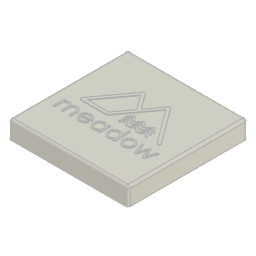
MeadowBox (Autodesk Fusion 360 design; units mm, degrees)
Autodesk Fusion 360 part; units mm, degrees
note: some values were not read from the file. Set by a fixed rule: which sketch regions a step uses.
(part 1 of 2)
sketch "Floor" plane through (0, 0, 0) normal (0, 0, 1) x (1, 0, 0) in component "Lid"
  line L0 (50, -50) -> (-50, -50)
  line L1 (-50, -50) -> (-50, 50)
  line L2 (-50, 50) -> (50, 50)
  line L3 (50, 50) -> (50, -50)
  line L4 (50, -50) -> (-50, 50) construction
  line L5 (-50, -50) -> (50, 50) construction
  line L6 (48, 48) -> (-48, 48)
  line L7 (-48, 48) -> (-48, -48)
  line L8 (-48, -48) -> (48, -48)
  line L9 (48, -48) -> (48, 48)
  line L10 (48, 48) -> (-48, -48) construction
  line L11 (-48, 48) -> (48, -48) construction
  dimension "d25" = 100
  dimension "d26" = 100
  dimension "d289" = 96
  dimension "d290" = 96
  constraint horizontal L0
  constraint perpendicular L0 L1
  constraint parallel L0 L2
  constraint parallel L1 L3
  constraint coincident L4 origin
  constraint coincident L5 origin
  constraint horizontal L6
  constraint perpendicular L6 L7
  constraint parallel L6 L8
  constraint parallel L7 L9
  constraint coincident L10 origin
  constraint coincident L11 origin
  measures "d25" distance of L1.end L2.end
  measures "d26" distance of L0.end L1.end
  measures "d289" distance of L7.end L8.end
  measures "d290" distance of L6.end L7.end
sketch "Floor (2)" plane through (0, 0, 0) normal (0, 0, 1) x (1, 0, 0) in component "Base"
  line L0 (50, -50) -> (-50, -50)
  line L1 (-50, -50) -> (-50, 50)
  line L2 (-50, 50) -> (50, 50)
  line L3 (50, 50) -> (50, -50)
  line L4 (50, -50) -> (-50, 50) construction
  line L5 (-50, -50) -> (50, 50) construction
  dimension "d109" = 100
  dimension "d110" = 100
  constraint horizontal L0
  constraint perpendicular L0 L1
  constraint parallel L0 L2
  constraint parallel L1 L3
  constraint coincident L4 origin
  constraint coincident L5 origin
  measures "d109" distance of L1.end L2.end
  measures "d110" distance of L0.end L1.end
extrude "Extrude19" add sketch "Floor (2)" along normal blind 18 makes body 1 in component "Base"
sketch "Walls" plane through (0, 0, 18) normal (0, 0, 1) x (-1, 0, 0) in component "Base"
  line L0 (-50, -50) -> (50, -50)
  line L1 (50, -50) -> (50, 50)
  line L2 (50, 50) -> (-50, 50)
  line L3 (-50, 50) -> (-50, -50)
  line L4 (-47, 47) -> (47, 47)
  line L5 (47, 47) -> (47, -47)
  line L6 (47, -47) -> (-47, -47)
  line L7 (-47, -47) -> (-47, 47)
  line L8 (-47, 47) -> (47, -47) construction
  line L9 (47, 47) -> (-47, -47) construction
  line L10 (48, 48) -> (-48, 48)
  line L11 (-48, 48) -> (-48, -48)
  line L12 (-48, -48) -> (48, -48)
  line L13 (48, -48) -> (48, 48)
  line L14 (48, 48) -> (-48, -48) construction
  line L15 (-48, 48) -> (48, -48) construction
  dimension "d252" = 94
  dimension "d253" = 94
  dimension "d256" = 96
  dimension "d257" = 96
  constraint horizontal L4
  constraint perpendicular L4 L5
  constraint parallel L4 L6
  constraint parallel L5 L7
  constraint coincident L8 origin
  constraint coincident L9 origin
  constraint horizontal L10
  constraint perpendicular L10 L11
  constraint parallel L10 L12
  constraint parallel L11 L13
  constraint coincident L14 origin
  constraint coincident L15 origin
  measures "d252" distance of L5.end L6.end
  measures "d253" distance of L4.end L5.end
  measures "d256" distance of L11.end L12.end
  measures "d257" distance of L10.end L11.end
extrude "Extrude20" cut sketch "Walls" against normal blind 16 contours L4 L5 L6 L7 bodies 1 in component "Base"
extrude "Extrude21" add sketch "Walls" along normal blind 0.4 contours L10 L11 L12 L13 bodies 1 in component "Base"
extrude "Extrude22" cut 1 faces at (47.6667, 15.6667, 18.4) along direction (0, 0, -1) blind 0.4 on bodies 1 bodies 1 in component "Base"
extrude "Extrude23" add sketch "Walls" along normal blind 4 contours L10 L11 L12 L13 bodies 1 in component "Base"
fillet "Fillet8" radius 2 8 edges at (50, 50, 9) (0, 50, 0) (-50, 50, 9) (50, 0, 0) (-50, 0, 0) (0, -50, 0) (50, -50, 9) (-50, -50, 9) on bodies 1 in component "Base"
chamfer "Chamfer4" distance 1 angle 70 4 edges at (0, 48, 22) (48, 0, 22) (-48, 0, 22) (0, -48, 22) measured on face at (47.6667, 15.6667, 22) measured on face at (47.6667, 15.6667, 22) measured on face at (47.6667, 15.6667, 22) measured on face at (47.6667, 15.6667, 22) on bodies 1 in component "Base"
sketch "Sketch18" plane through (0, 0, 2) normal (0, 0, 1) x (-1, 0, 0) in component "Base"
  line L0 (-47, -47) -> (47, -47)
  line L1 (47, -47) -> (47, 47)
  line L2 (47, 47) -> (-47, 47)
  line L3 (-47, 47) -> (-47, -47)
  line L4 (0, -47) -> (0, 47) construction
  line L5 (47, 0) -> (-47, 0) construction
  line L6 (-41, -3) -> (-47, -3)
  line L7 (-47, -3) -> (-47, 3)
  line L8 (-47, 3) -> (-41, 3)
  line L9 (-41, 3) -> (-41, -3)
  line L10 (-44, -3) -> (-44, 3) construction
  line L11 (-41, 0) -> (-47, 0) construction
  line L12 (41, 3) -> (47, 3)
  line L13 (47, 3) -> (47, -3)
  line L14 (47, -3) -> (41, -3)
  line L15 (44, -3) -> (44, 3) construction
  line L16 (47, 0) -> (41, 0) construction
  line L17 (41, -3) -> (41, 3)
  line L18 (0, -47) -> (0, 47) construction
  line L19 (47, 0) -> (-47, 0) construction
  line L20 (3, -47) -> (-3, -47)
  line L21 (-3, -47) -> (-3, -41)
  line L22 (-3, -41) -> (3, -41)
  line L23 (3, -41) -> (3, -47)
  line L24 (3, 41) -> (-3, 41)
  line L25 (-3, 41) -> (-3, 47)
  line L26 (-3, 47) -> (3, 47)
  line L27 (3, 47) -> (3, 41)
  line L28 (0, -47) -> (0, -41) construction
  line L29 (0, 41) -> (0, 47) construction
  dimension "d267" = 6
  dimension "d268" = 6
  dimension "d269" = 6
  dimension "d270" = 6
  dimension "d271" = 6
  dimension "d272" = 6
  dimension "d273" = 6
  dimension "d274" = 6
  constraint midpoint L0 L4.start
  constraint midpoint L2 L4.end
  constraint midpoint L1 L5.start
  constraint midpoint L3 L5.end
  constraint horizontal L6
  constraint vertical L7
  constraint horizontal L8
  constraint vertical L9
  constraint midpoint L6 L10.start
  constraint midpoint L8 L10.end
  constraint midpoint L9 L11.start
  constraint midpoint L7 L5.end
  constraint horizontal L14
  constraint vertical L17
  constraint horizontal L12
  constraint vertical L13
  constraint midpoint L15.start L14
  constraint midpoint L15.end L12
  constraint midpoint L5.start L13
  constraint midpoint L16.end L17
  constraint coincident L5.start L13
  constraint collinear L16 L19
  constraint collinear L5 L11
  constraint collinear L3 L7
  constraint horizontal L20
  constraint vertical L21
  constraint horizontal L22
  constraint vertical L23
  constraint horizontal L24
  constraint vertical L25
  constraint horizontal L26
  constraint vertical L27
  constraint collinear L0 L20
  constraint collinear L2 L26
  constraint midpoint L20 L4.start
  constraint midpoint L22 L28.end
  constraint midpoint L24 L29.start
  constraint midpoint L26 L4.end
  constraint collinear L18 L29
  constraint collinear L18 L28
  measures "d267" distance of L6.start L6.end
  measures "d268" distance of L6.start L8.end
  measures "d269" distance of L14.end L13.end
  measures "d270" distance of L12.end L13.end
  measures "d271" distance of L20.start L20.end
  measures "d272" distance of L20.start L22.end
  measures "d273" distance of L24.start L24.end
  measures "d274" distance of L24.start L26.end
extrude "Extrude24" add sketch "Sketch18" along normal blind 6 contours L0 L20 L21 L22 L23 | L3 L6 L7 L8 L9 | L1 L12 L13 L14 L17 | L2 L24 L25 L26 L27 bodies 1 in component "Base"
extrude "Extrude25" add 1 faces at (45, 1, 8) along direction (0, 0, 1) blind 3 on bodies 1 bodies 1 in component "Base"
extrude "Extrude26" cut 1 faces at (45, 1, 11) along direction (0, 0, -1) blind 3 on bodies 1 bodies 1 in component "Base"
sketch "Sketch20" plane through (0, 47, 0) normal (0, -1, 0) x (1, 0, 0) in component "Base"
  line L0 (3, 8) -> (3, 2)
  line L1 (3, 2) -> (47, 2)
  line L2 (47, 2) -> (47, 22)
  line L3 (47, 22) -> (-47, 22)
  line L4 (-47, 22) -> (-47, 2)
  line L5 (-47, 2) -> (-3, 2)
  line L6 (-3, 2) -> (-3, 8)
  line L7 (-3, 8) -> (3, 8)
  line L8 (23, 22) -> (36, 22)
  line L9 (36, 22) -> (36, 11)
  line L10 (36, 11) -> (23, 11)
  line L11 (23, 11) -> (23, 22)
  dimension "d281" = 13
  dimension "d282" = 11
  dimension "d283" = 9
  dimension "d284" = 11
  constraint horizontal L8
  constraint vertical L9
  constraint horizontal L10
  constraint vertical L11
  measures "d281" distance of L8.start L8.end
  measures "d282" distance of L8.start L10.end
  measures "d283" distance of L1 L10
  measures "d284" distance of L2 L9
extrude "Extrude35" add sketch "Floor" along normal blind 15 separate body contours L0 L1 L2 L3 | L6 L7 L8 L9 makes body 2 in component "Lid"
extrude "Extrude36" cut sketch "Floor" along normal blind 13 contours L6 L7 L8 L9 bodies 2 in component "Lid"
fillet "Fillet8'" radius 2 8 edges at (50, -50, 7.5) (50, 0, 15) (0, -50, 15) (50, 50, 7.5) (0, 50, 15) (-50, 50, 7.5) (-50, 0, 15) (-50, -50, 7.5) on bodies 2 in component "Lid"
sketch "Sketch13" plane through (0, 50, 0) normal (0, 1, 0) x (-1, 0, 0) in component "Lid"
  line L0 (48, 0) -> (48, 13)
  line L1 (48, 13) -> (-48, 13)
  line L2 (-48, 13) -> (-48, 0)
  line L3 (-48, 0) -> (48, 0)
  line L4 (-36, 2) -> (-23, 2)
  line L5 (-23, 2) -> (-23, 0)
  line L6 (-23, 0) -> (-36, 0)
  line L7 (-36, 0) -> (-36, 2)
  line L8 (50, 0) -> (-50, 0)
  dimension "d306" = 13
  dimension "d307" = 2
  dimension "d308" = 12
  constraint horizontal L4
  constraint vertical L5
  constraint horizontal L6
  constraint vertical L7
  constraint collinear L6 L8
  measures "d306" distance of L4.start L4.end
  measures "d307" distance of L4.start L6.end
  measures "d308" distance of L2 L7
extrude "Extrude28" cut sketch "Sketch20" against normal blind 3 contours L3 L8 L9 L10 L11 bodies 1 in component "Base"
extrude "Extrude37" cut sketch "Sketch13" against normal blind 2 contours L3 L4 L5 L6 L7 L8 bodies 2 in component "Lid"
sketch "Sketch14" plane through (0, 0, 15) normal (0, 0, 1) x (-1, 0, 0) in component "Lid"
  line L0 (-48, -48) -> (48, -48)
  line L1 (48, -48) -> (48, 48)
  line L2 (48, 48) -> (-48, 48)
  line L3 (-48, 48) -> (-48, -48)
  line L4 (25.0801, 17.3069) -> (25.0801, 22.7705)
  line L5 (25.0801, 22.7705) -> (26.3528, 22.7705)
  line L6 (26.3528, 22.7705) -> (26.3528, 17.3333)
  spline S0 degree 3 poles (26.3528, 17.3333) (26.3528, 16.9685) (26.4246, 16.6073) (26.5642, 16.2702) knots 0 0 0 0 1 1 1 1
  spline S1 degree 3 poles (26.5642, 16.2702) (26.7038, 15.9332) (26.9085, 15.6268) (27.1665, 15.3688) knots 0 0 0 0 1 1 1 1
  spline S2 degree 3 poles (27.1665, 15.3688) (27.4244, 15.1108) (27.7307, 14.9063) (28.0677, 14.7666) knots 0 0 0 0 1 1 1 1
  spline S3 degree 3 poles (28.0677, 14.7666) (28.4048, 14.6272) (28.7661, 14.5552) (29.1309, 14.5552) knots 0 0 0 0 1 1 1 1
  spline S4 degree 3 poles (29.1309, 14.5552) (29.4957, 14.5552) (29.857, 14.6272) (30.194, 14.7666) knots 0 0 0 0 1 1 1 1
  spline S5 degree 3 poles (30.194, 14.7666) (30.5311, 14.9063) (30.8373, 15.1108) (31.0953, 15.3688) knots 0 0 0 0 1 1 1 1
  spline S6 degree 3 poles (31.0953, 15.3688) (31.3533, 15.6268) (31.5579, 15.9332) (31.6975, 16.2702) knots 0 0 0 0 1 1 1 1
  spline S7 degree 3 poles (31.6975, 16.2702) (31.8372, 16.6073) (31.909, 16.9685) (31.909, 17.3333) knots 0 0 0 0 1 1 1 1
  line L7 (31.909, 17.3333) -> (31.909, 22.7599)
  line L8 (31.909, 22.7599) -> (33.1605, 22.7599)
  line L9 (33.1605, 22.7599) -> (33.1605, 17.3333)
  spline S8 degree 3 poles (33.1605, 17.3333) (33.149, 16.96) (33.2126, 16.5883) (33.3475, 16.2401) knots 0 0 0 0 1 1 1 1
  spline S9 degree 3 poles (33.3475, 16.2401) (33.4824, 15.8919) (33.6859, 15.5741) (33.9458, 15.3061) knots 0 0 0 0 1 1 1 1
  spline S10 degree 3 poles (33.9458, 15.3061) (34.2058, 15.0381) (34.517, 14.8248) (34.8609, 14.6793) knots 0 0 0 0 1 1 1 1
  spline S11 degree 3 poles (34.8609, 14.6793) (35.2048, 14.5338) (35.5744, 14.4586) (35.9479, 14.4586) knots 0 0 0 0 1 1 1 1
  spline S12 degree 3 poles (35.9479, 14.4586) (36.3213, 14.4586) (36.691, 14.5338) (37.0349, 14.6793) knots 0 0 0 0 1 1 1 1
  spline S13 degree 3 poles (37.0349, 14.6793) (37.3788, 14.8248) (37.69, 15.0381) (37.9499, 15.3061) knots 0 0 0 0 1 1 1 1
  spline S14 degree 3 poles (37.9499, 15.3061) (38.2099, 15.5741) (38.4134, 15.8919) (38.5483, 16.2401) knots 0 0 0 0 1 1 1 1
  spline S15 degree 3 poles (38.5483, 16.2401) (38.6832, 16.5883) (38.7468, 16.96) (38.7353, 17.3333) knots 0 0 0 0 1 1 1 1
  line L10 (38.7353, 17.3333) -> (38.7353, 22.7599)
  line L11 (38.7353, 22.7599) -> (39.9682, 22.7599)
  line L12 (39.9682, 22.7599) -> (39.9682, 13.4995)
  line L13 (39.9682, 13.4995) -> (38.7353, 13.4995)
  line L14 (38.7353, 13.4995) -> (38.7353, 14.8701)
  spline S16 degree 3 poles (38.7353, 14.8701) (38.3569, 14.3599) (37.8558, 13.9538) (37.2785, 13.6892) knots 0 0 0 0 1 1 1 1
  spline S17 degree 3 poles (37.2785, 13.6892) (36.7012, 13.4244) (36.0664, 13.3098) (35.433, 13.3561) knots 0 0 0 0 1 1 1 1
  spline S18 degree 3 poles (35.433, 13.3561) (34.7996, 13.4022) (34.1881, 13.6077) (33.6553, 13.9533) knots 0 0 0 0 1 1 1 1
  spline S19 degree 3 poles (33.6553, 13.9533) (33.1225, 14.2988) (32.6856, 14.7735) (32.3853, 15.3331) knots 0 0 0 0 1 1 1 1
  spline S20 degree 3 poles (32.3853, 15.3331) (32.0415, 14.7192) (31.5363, 14.2112) (30.9243, 13.8644) knots 0 0 0 0 1 1 1 1
  spline S21 degree 3 poles (30.9243, 13.8644) (30.3124, 13.5172) (29.6171, 13.3445) (28.9139, 13.3646) knots 0 0 0 0 1 1 1 1
  spline S22 degree 3 poles (28.9139, 13.3646) (26.7258, 13.3646) (25.0801, 15.1029) (25.0801, 17.3069) knots 0 0 0 0 1 1 1 1
  line L15 (14.0894, 19.3442) -> (13.031, 19.7146)
  spline S23 degree 3 poles (13.031, 19.7146) (13.4099, 20.6337) (14.0527, 21.4198) (14.8783, 21.9736) knots 0 0 0 0 1 1 1 1
  spline S24 degree 3 poles (14.8783, 21.9736) (15.7038, 22.5276) (16.675, 22.8242) (17.6692, 22.8261) knots 0 0 0 0 1 1 1 1
  spline S25 degree 3 poles (17.6692, 22.8261) (18.7049, 22.816) (19.711, 22.4795) (20.5442, 21.8641) knots 0 0 0 0 1 1 1 1
  spline S26 degree 3 poles (20.5442, 21.8641) (21.3775, 21.2489) (21.9954, 20.3866) (22.31, 19.3997) knots 0 0 0 0 1 1 1 1
  spline S27 degree 3 poles (22.31, 19.3997) (22.4352, 18.97) (22.4976, 18.5245) (22.4952, 18.0768) knots 0 0 0 0 1 1 1 1
  spline S28 degree 3 poles (22.4952, 18.0768) (22.4943, 16.8518) (22.0265, 15.6731) (21.187, 14.7806) knots 0 0 0 0 1 1 1 1
  spline S29 degree 3 poles (21.187, 14.7806) (20.3475, 13.8885) (19.1995, 13.3495) (17.9767, 13.2741) knots 0 0 0 0 1 1 1 1
  spline S30 degree 3 poles (17.9767, 13.2741) (16.7539, 13.1984) (15.5483, 13.5919) (14.6053, 14.374) knots 0 0 0 0 1 1 1 1
  spline S31 degree 3 poles (14.6053, 14.374) (13.6624, 15.1563) (13.053, 16.2684) (12.9014, 17.4841) knots 0 0 0 0 1 1 1 1
  spline S32 degree 3 poles (12.9014, 17.4841) (12.8868, 17.5635) (12.8805, 17.6442) (12.8829, 17.7249) knots 0 0 0 0 1 1 1 1
  line L16 (12.8829, 17.7249) -> (21.0664, 19.1854)
  spline S33 degree 3 poles (21.0664, 19.1854) (20.849, 19.9143) (20.4018, 20.5533) (19.7915, 21.0073) knots 0 0 0 0 1 1 1 1
  spline S34 degree 3 poles (19.7915, 21.0073) (19.1811, 21.4614) (18.4404, 21.7058) (17.6798, 21.7043) knots 0 0 0 0 1 1 1 1
  spline S35 degree 3 poles (17.6798, 21.7043) (15.9229, 21.6963) (14.5207, 20.5083) (14.0894, 19.3442) knots 0 0 0 0 1 1 1 1
  spline S36 degree 3 poles (21.2728, 17.7567) (21.2728, 17.8678) (21.2543, 17.9974) (21.2543, 18.1826) knots 0 0 0 0 1 1 1 1
  line L17 (21.2543, 18.1826) -> (14.2958, 16.9418)
  spline S37 degree 3 poles (14.2958, 16.9418) (14.5336, 16.202) (15.0008, 15.5574) (15.6297, 15.101) knots 0 0 0 0 1 1 1 1
  spline S38 degree 3 poles (15.6297, 15.101) (16.2587, 14.6449) (17.0166, 14.401) (17.7935, 14.4044) knots 0 0 0 0 1 1 1 1
  spline S39 degree 3 poles (17.7935, 14.4044) (18.6884, 14.4216) (19.5438, 14.7759) (20.1889, 15.3963) knots 0 0 0 0 1 1 1 1
  spline S40 degree 3 poles (20.1889, 15.3963) (20.8339, 16.0168) (21.221, 16.8579) (21.2728, 17.7514) knots 0 0 0 0 1 1 1 1
  line L18 (21.2728, 17.7514) -> (21.2728, 17.7567)
  line L19 (1.0586, 13.5101) -> (1.0586, 22.7705)
  line L20 (1.0586, 22.7705) -> (2.2916, 22.7705)
  line L21 (2.2916, 22.7705) -> (2.2916, 21.2703)
  spline S41 degree 3 poles (2.2916, 21.2703) (2.7475, 21.7887) (3.3089, 22.2038) (3.9381, 22.4882) knots 0 0 0 0 1 1 1 1
  spline S42 degree 3 poles (3.9381, 22.4882) (4.5673, 22.7724) (5.2499, 22.9192) (5.9402, 22.9187) knots 0 0 0 0 1 1 1 1
  spline S43 degree 3 poles (5.9402, 22.9187) (6.7387, 22.9123) (7.5229, 22.706) (8.2212, 22.3183) knots 0 0 0 0 1 1 1 1
  spline S44 degree 3 poles (8.2212, 22.3183) (8.9194, 21.9307) (9.5094, 21.3743) (9.937, 20.6999) knots 0 0 0 0 1 1 1 1
  spline S45 degree 3 poles (9.937, 20.6999) (10.3648, 20.0257) (10.6167, 19.2547) (10.6699, 18.4581) knots 0 0 0 0 1 1 1 1
  spline S46 degree 3 poles (10.6699, 18.4581) (10.7228, 17.6612) (10.5754, 16.8637) (10.2407, 16.1387) knots 0 0 0 0 1 1 1 1
  spline S47 degree 3 poles (10.2407, 16.1387) (9.9063, 15.4135) (9.3954, 14.7838) (8.7548, 14.307) knots 0 0 0 0 1 1 1 1
  spline S48 degree 3 poles (8.7548, 14.307) (8.114, 13.8302) (7.3642, 13.5217) (6.5736, 13.4096) knots 0 0 0 0 1 1 1 1
  spline S49 degree 3 poles (6.5736, 13.4096) (5.7828, 13.2974) (4.9768, 13.385) (4.2286, 13.6646) knots 0 0 0 0 1 1 1 1
  spline S50 degree 3 poles (4.2286, 13.6646) (3.4806, 13.9443) (2.8147, 14.407) (2.2916, 15.0103) knots 0 0 0 0 1 1 1 1
  line L22 (2.2916, 15.0103) -> (2.2916, 13.5101)
  line L23 (2.2916, 13.5101) -> (1.0586, 13.5101)
  spline S51 degree 3 poles (2.3286, 18.1403) (2.3307, 17.4283) (2.544, 16.7327) (2.9411, 16.1419) knots 0 0 0 0 1 1 1 1
  spline S52 degree 3 poles (2.9411, 16.1419) (3.3385, 15.5508) (3.9021, 15.091) (4.5606, 14.8203) knots 0 0 0 0 1 1 1 1
  spline S53 degree 3 poles (4.5606, 14.8203) (5.2195, 14.5497) (5.9434, 14.4803) (6.6416, 14.6211) knots 0 0 0 0 1 1 1 1
  spline S54 degree 3 poles (6.6416, 14.6211) (7.3396, 14.7618) (7.9801, 15.1063) (8.4823, 15.6112) knots 0 0 0 0 1 1 1 1
  spline S55 degree 3 poles (8.4823, 15.6112) (8.9847, 16.116) (9.3258, 16.7584) (9.4631, 17.4572) knots 0 0 0 0 1 1 1 1
  spline S56 degree 3 poles (9.4631, 17.4572) (9.6002, 18.1559) (9.5271, 18.8796) (9.253, 19.5368) knots 0 0 0 0 1 1 1 1
  spline S57 degree 3 poles (9.253, 19.5368) (8.9792, 20.194) (8.5164, 20.7555) (7.9232, 21.1497) knots 0 0 0 0 1 1 1 1
  spline S58 degree 3 poles (7.9232, 21.1497) (7.3303, 21.5439) (6.6337, 21.7535) (5.9217, 21.7519) knots 0 0 0 0 1 1 1 1
  spline S59 degree 3 poles (5.9217, 21.7519) (5.4473, 21.7558) (4.9766, 21.6648) (4.5376, 21.4846) knots 0 0 0 0 1 1 1 1
  spline S60 degree 3 poles (4.5376, 21.4846) (4.099, 21.3042) (3.7005, 21.038) (3.3658, 20.7017) knots 0 0 0 0 1 1 1 1
  spline S61 degree 3 poles (3.3658, 20.7017) (3.0311, 20.3652) (2.7668, 19.9654) (2.5887, 19.5257) knots 0 0 0 0 1 1 1 1
  spline S62 degree 3 poles (2.5887, 19.5257) (2.4106, 19.0857) (2.3223, 18.6147) (2.3286, 18.1403) knots 0 0 0 0 1 1 1 1
  line L24 (-11.3424, 8.991) -> (-11.3424, 22.7705)
  line L25 (-11.3424, 22.7705) -> (-10.1094, 22.7705)
  line L26 (-10.1094, 22.7705) -> (-10.1094, 21.2703)
  spline S63 degree 3 poles (-10.1094, 21.2703) (-9.653, 21.7884) (-9.0919, 22.2033) (-8.4627, 22.4874) knots 0 0 0 0 1 1 1 1
  spline S64 degree 3 poles (-8.4627, 22.4874) (-7.8335, 22.7716) (-7.1511, 22.9187) (-6.4608, 22.9187) knots 0 0 0 0 1 1 1 1
  spline S65 degree 3 poles (-6.4608, 22.9187) (-5.6623, 22.9123) (-4.8781, 22.706) (-4.1799, 22.3183) knots 0 0 0 0 1 1 1 1
  spline S66 degree 3 poles (-4.1799, 22.3183) (-3.4816, 21.9307) (-2.8919, 21.3743) (-2.464, 20.6999) knots 0 0 0 0 1 1 1 1
  spline S67 degree 3 poles (-2.464, 20.6999) (-2.0362, 20.0257) (-1.7843, 19.2547) (-1.7311, 18.4581) knots 0 0 0 0 1 1 1 1
  spline S68 degree 3 poles (-1.7311, 18.4581) (-1.6782, 17.6612) (-1.8256, 16.8637) (-2.1603, 16.1387) knots 0 0 0 0 1 1 1 1
  spline S69 degree 3 poles (-2.1603, 16.1387) (-2.4947, 15.4135) (-3.0056, 14.7838) (-3.6465, 14.307) knots 0 0 0 0 1 1 1 1
  spline S70 degree 3 poles (-3.6465, 14.307) (-4.287, 13.8302) (-5.0368, 13.5217) (-5.8274, 13.4096) knots 0 0 0 0 1 1 1 1
  spline S71 degree 3 poles (-5.8274, 13.4096) (-6.6183, 13.2974) (-7.4244, 13.385) (-8.1724, 13.6646) knots 0 0 0 0 1 1 1 1
  spline S72 degree 3 poles (-8.1724, 13.6646) (-8.9204, 13.9443) (-9.5864, 14.407) (-10.1094, 15.0103) knots 0 0 0 0 1 1 1 1
  line L27 (-10.1094, 15.0103) -> (-10.1094, 8.991)
  line L28 (-10.1094, 8.991) -> (-11.3424, 8.991)
  spline S73 degree 3 poles (-10.0698, 18.1403) (-10.0676, 17.4281) (-9.8544, 16.7325) (-9.457, 16.1414) knots 0 0 0 0 1 1 1 1
  spline S74 degree 3 poles (-9.457, 16.1414) (-9.0596, 15.5506) (-8.4957, 15.0907) (-7.8369, 14.8201) knots 0 0 0 0 1 1 1 1
  spline S75 degree 3 poles (-7.8369, 14.8201) (-7.1784, 14.5494) (-6.454, 14.4803) (-5.756, 14.6211) knots 0 0 0 0 1 1 1 1
  spline S76 degree 3 poles (-5.756, 14.6211) (-5.0577, 14.7621) (-4.4172, 15.1071) (-3.915, 15.6122) knots 0 0 0 0 1 1 1 1
  spline S77 degree 3 poles (-3.915, 15.6122) (-3.4128, 16.1173) (-3.0718, 16.7597) (-2.935, 17.4587) knots 0 0 0 0 1 1 1 1
  spline S78 degree 3 poles (-2.935, 17.4587) (-2.7982, 18.1578) (-2.8715, 18.8814) (-3.1461, 19.5386) knots 0 0 0 0 1 1 1 1
  spline S79 degree 3 poles (-3.1461, 19.5386) (-3.4205, 20.1959) (-3.8838, 20.757) (-4.477, 21.151) knots 0 0 0 0 1 1 1 1
  spline S80 degree 3 poles (-4.477, 21.151) (-5.0704, 21.5447) (-5.7671, 21.754) (-6.4794, 21.7519) knots 0 0 0 0 1 1 1 1
  spline S81 degree 3 poles (-6.4794, 21.7519) (-6.9538, 21.7558) (-7.4242, 21.6648) (-7.8629, 21.4846) knots 0 0 0 0 1 1 1 1
  spline S82 degree 3 poles (-7.8629, 21.4846) (-8.3018, 21.3042) (-8.7, 21.038) (-9.0344, 20.7015) knots 0 0 0 0 1 1 1 1
  spline S83 degree 3 poles (-9.0344, 20.7015) (-9.3689, 20.3652) (-9.6327, 19.9651) (-9.8105, 19.5254) knots 0 0 0 0 1 1 1 1
  spline S84 degree 3 poles (-9.8105, 19.5254) (-9.9883, 19.0857) (-10.0764, 18.6147) (-10.0698, 18.1403) knots 0 0 0 0 1 1 1 1
  spline S85 degree 3 poles (-14.0359, 18.1403) (-14.0263, 17.1838) (-14.3015, 16.2462) (-14.8259, 15.4463) knots 0 0 0 0 1 1 1 1
  spline S86 degree 3 poles (-14.8259, 15.4463) (-15.3503, 14.6465) (-16.1009, 14.0205) (-16.9817, 13.648) knots 0 0 0 0 1 1 1 1
  spline S87 degree 3 poles (-16.9817, 13.648) (-17.8628, 13.2752) (-18.8346, 13.1728) (-19.7739, 13.3537) knots 0 0 0 0 1 1 1 1
  spline S88 degree 3 poles (-19.7739, 13.3537) (-20.7131, 13.5344) (-21.5775, 13.9903) (-22.2573, 14.6634) knots 0 0 0 0 1 1 1 1
  spline S89 degree 3 poles (-22.2573, 14.6634) (-22.9367, 15.3363) (-23.4013, 16.1962) (-23.5913, 17.1336) knots 0 0 0 0 1 1 1 1
  spline S90 degree 3 poles (-23.5913, 17.1336) (-23.7815, 18.071) (-23.6886, 19.0439) (-23.3248, 19.9284) knots 0 0 0 0 1 1 1 1
  spline S91 degree 3 poles (-23.3248, 19.9284) (-22.961, 20.8129) (-22.3424, 21.5696) (-21.5479, 22.1019) knots 0 0 0 0 1 1 1 1
  spline S92 degree 3 poles (-21.5479, 22.1019) (-20.7534, 22.6343) (-19.8183, 22.9187) (-18.8619, 22.9187) knots 0 0 0 0 1 1 1 1
  spline S93 degree 3 poles (-18.8619, 22.9187) (-18.2308, 22.9235) (-17.6048, 22.8036) (-17.0204, 22.5657) knots 0 0 0 0 1 1 1 1
  spline S94 degree 3 poles (-17.0204, 22.5657) (-16.4356, 22.3281) (-15.9038, 21.977) (-15.4553, 21.5328) knots 0 0 0 0 1 1 1 1
  spline S95 degree 3 poles (-15.4553, 21.5328) (-15.0069, 21.0888) (-14.6505, 20.5605) (-14.4068, 19.9784) knots 0 0 0 0 1 1 1 1
  spline S96 degree 3 poles (-14.4068, 19.9784) (-14.1634, 19.396) (-14.0372, 18.7713) (-14.0359, 18.1403) knots 0 0 0 0 1 1 1 1
  spline S97 degree 3 poles (-22.4708, 18.1403) (-22.4665, 17.4312) (-22.2525, 16.7391) (-21.8553, 16.1514) knots 0 0 0 0 1 1 1 1
  spline S98 degree 3 poles (-21.8553, 16.1514) (-21.4582, 15.5638) (-20.8962, 15.1069) (-20.2398, 14.8383) knots 0 0 0 0 1 1 1 1
  spline S99 degree 3 poles (-20.2398, 14.8383) (-19.5834, 14.5698) (-18.8621, 14.5018) (-18.1671, 14.6428) knots 0 0 0 0 1 1 1 1
  spline S100 degree 3 poles (-18.1671, 14.6428) (-17.472, 14.7835) (-16.8341, 15.1272) (-16.3343, 15.6302) knots 0 0 0 0 1 1 1 1
  spline S101 degree 3 poles (-16.3343, 15.6302) (-15.8342, 16.1332) (-15.4942, 16.7729) (-15.3574, 17.4688) knots 0 0 0 0 1 1 1 1
  spline S102 degree 3 poles (-15.3574, 17.4688) (-15.2207, 18.1647) (-15.2929, 18.8854) (-15.5654, 19.5402) knots 0 0 0 0 1 1 1 1
  spline S103 degree 3 poles (-15.5654, 19.5402) (-15.8377, 20.1951) (-16.2978, 20.7547) (-16.8878, 21.1484) knots 0 0 0 0 1 1 1 1
  spline S104 degree 3 poles (-16.8878, 21.1484) (-17.4778, 21.5418) (-18.171, 21.7519) (-18.8804, 21.7519) knots 0 0 0 0 1 1 1 1
  spline S105 degree 3 poles (-18.8804, 21.7519) (-19.354, 21.7532) (-19.8234, 21.6606) (-20.261, 21.4794) knots 0 0 0 0 1 1 1 1
  spline S106 degree 3 poles (-20.261, 21.4794) (-20.6986, 21.2981) (-21.0957, 21.0319) (-21.4299, 20.6959) knots 0 0 0 0 1 1 1 1
  spline S107 degree 3 poles (-21.4299, 20.6959) (-21.7638, 20.3599) (-22.0279, 19.9612) (-22.2065, 19.5225) knots 0 0 0 0 1 1 1 1
  spline S108 degree 3 poles (-22.2065, 19.5225) (-22.385, 19.0838) (-22.475, 18.6139) (-22.4708, 18.1403) knots 0 0 0 0 1 1 1 1
  line L29 (-39.3988, 13.5101) -> (-36.0889, 22.7705)
  line L30 (-36.0889, 22.7705) -> (-34.8533, 22.7705)
  line L31 (-34.8533, 22.7705) -> (-32.2074, 15.1399)
  line L32 (-32.2074, 15.1399) -> (-29.5616, 22.7705)
  line L33 (-29.5616, 22.7705) -> (-28.326, 22.7705)
  line L34 (-28.326, 22.7705) -> (-25.0346, 13.5101)
  line L35 (-25.0346, 13.5101) -> (-26.2702, 13.5101)
  line L36 (-26.2702, 13.5101) -> (-28.961, 21.0375)
  line L37 (-28.961, 21.0375) -> (-31.6545, 13.4995)
  line L38 (-31.6545, 13.4995) -> (-32.7789, 13.4995)
  line L39 (-32.7789, 13.4995) -> (-35.4724, 21.0375)
  line L40 (-35.4724, 21.0375) -> (-38.1659, 13.4995)
  line L41 (-38.1659, 13.4995) -> (-39.3988, 13.5101)
  line L42 (11.2689, 6.8267) -> (32.4355, 6.8267)
  spline S109 degree 3 poles (32.4355, 6.8267) (32.6702, 6.8267) (32.9002, 6.7616) (33.0997, 6.6381) knots 0 0 0 0 1 1 1 1
  spline S110 degree 3 poles (33.0997, 6.6381) (33.2993, 6.5148) (33.4606, 6.338) (33.5653, 6.1282) knots 0 0 0 0 1 1 1 1
  spline S111 degree 3 poles (33.5653, 6.1282) (33.6691, 5.9184) (33.7133, 5.684) (33.6933, 5.4509) knots 0 0 0 0 1 1 1 1
  spline S112 degree 3 poles (33.6933, 5.4509) (33.6732, 5.2175) (33.5896, 4.9945) (33.4515, 4.8053) knots 0 0 0 0 1 1 1 1
  line L43 (33.4515, 4.8053) -> (11.9542, -24.3968)
  spline S113 degree 3 poles (11.9542, -24.3968) (11.8367, -24.5571) (11.6827, -24.6874) (11.5054, -24.7771) knots 0 0 0 0 1 1 1 1
  spline S114 degree 3 poles (11.5054, -24.7771) (11.3279, -24.8668) (11.1316, -24.9132) (10.9329, -24.9127) knots 0 0 0 0 1 1 1 1
  spline S115 degree 3 poles (10.9329, -24.9127) (10.7352, -24.912) (10.5408, -24.8649) (10.3648, -24.7753) knots 0 0 0 0 1 1 1 1
  spline S116 degree 3 poles (10.3648, -24.7753) (10.1889, -24.6857) (10.0362, -24.556) (9.9195, -24.3968) knots 0 0 0 0 1 1 1 1
  line L44 (9.9195, -24.3968) -> (-0.6638, -10.0246)
  spline S117 degree 3 poles (-0.6638, -10.0246) (-0.8628, -9.7531) (-0.9467, -9.4141) (-0.8969, -9.0812) knots 0 0 0 0 1 1 1 1
  spline S118 degree 3 poles (-0.8969, -9.0812) (-0.8474, -8.7483) (-0.6686, -8.4484) (-0.3992, -8.2466) knots 0 0 0 0 1 1 1 1
  spline S119 degree 3 poles (-0.3992, -8.2466) (-0.2661, -8.147) (-0.1145, -8.0748) (0.0466, -8.0342) knots 0 0 0 0 1 1 1 1
  spline S120 degree 3 poles (0.0466, -8.0342) (0.2077, -7.9936) (0.3752, -7.9854) (0.5398, -8.01) knots 0 0 0 0 1 1 1 1
  spline S121 degree 3 poles (0.5398, -8.01) (0.7041, -8.0346) (0.862, -8.0915) (1.0041, -8.1776) knots 0 0 0 0 1 1 1 1
  spline S122 degree 3 poles (1.0041, -8.1776) (1.1465, -8.2636) (1.27, -8.377) (1.3682, -8.5112) knots 0 0 0 0 1 1 1 1
  line L45 (1.3682, -8.5112) -> (10.9329, -21.5049)
  line L46 (10.9329, -21.5049) -> (29.9193, 4.2841)
  line L47 (29.9193, 4.2841) -> (11.2689, 4.2841)
  spline S123 degree 3 poles (11.2689, 4.2841) (10.9416, 4.2989) (10.6328, 4.4394) (10.4066, 4.6762) knots 0 0 0 0 1 1 1 1
  spline S124 degree 3 poles (10.4066, 4.6762) (10.1804, 4.913) (10.0542, 5.2279) (10.0542, 5.5554) knots 0 0 0 0 1 1 1 1
  spline S125 degree 3 poles (10.0542, 5.5554) (10.0542, 5.883) (10.1804, 6.1978) (10.4066, 6.4346) knots 0 0 0 0 1 1 1 1
  spline S126 degree 3 poles (10.4066, 6.4346) (10.6328, 6.6714) (10.9416, 6.8119) (11.2689, 6.8267) knots 0 0 0 0 1 1 1 1
  spline S127 degree 3 poles (-31.7206, 6.8267) (-31.523, 6.827) (-31.3277, 6.7807) (-31.1512, 6.6915) knots 0 0 0 0 1 1 1 1
  spline S128 degree 3 poles (-31.1512, 6.6915) (-30.9747, 6.6024) (-30.8218, 6.4727) (-30.7046, 6.3134) knots 0 0 0 0 1 1 1 1
  line L48 (-30.7046, 6.3134) -> (-10.2259, -21.5049)
  line L49 (-10.2259, -21.5049) -> (10.2529, 6.3134)
  spline S129 degree 3 poles (10.2529, 6.3134) (10.3513, 6.4473) (10.4751, 6.5606) (10.6172, 6.6463) knots 0 0 0 0 1 1 1 1
  spline S130 degree 3 poles (10.6172, 6.6463) (10.7596, 6.732) (10.9173, 6.7889) (11.0816, 6.8135) knots 0 0 0 0 1 1 1 1
  spline S131 degree 3 poles (11.0816, 6.8135) (11.2459, 6.8381) (11.4134, 6.8299) (11.5745, 6.7897) knots 0 0 0 0 1 1 1 1
  spline S132 degree 3 poles (11.5745, 6.7897) (11.7356, 6.7492) (11.887, 6.6772) (12.0203, 6.578) knots 0 0 0 0 1 1 1 1
  spline S133 degree 3 poles (12.0203, 6.578) (12.2902, 6.3767) (12.4696, 6.0766) (12.5191, 5.7435) knots 0 0 0 0 1 1 1 1
  spline S134 degree 3 poles (12.5191, 5.7435) (12.5688, 5.4104) (12.4844, 5.0712) (12.2849, 4.8) knots 0 0 0 0 1 1 1 1
  line L50 (12.2849, 4.8) -> (-9.2125, -24.3967)
  spline S135 degree 3 poles (-9.2125, -24.3967) (-9.3292, -24.5564) (-9.4818, -24.6863) (-9.6583, -24.7758) knots 0 0 0 0 1 1 1 1
  spline S136 degree 3 poles (-9.6583, -24.7758) (-9.8345, -24.8653) (-10.0295, -24.912) (-10.2272, -24.912) knots 0 0 0 0 1 1 1 1
  spline S137 degree 3 poles (-10.2272, -24.912) (-10.4248, -24.912) (-10.6198, -24.8653) (-10.7963, -24.7758) knots 0 0 0 0 1 1 1 1
  spline S138 degree 3 poles (-10.7963, -24.7758) (-10.9725, -24.6863) (-11.1252, -24.5564) (-11.2419, -24.3967) knots 0 0 0 0 1 1 1 1
  line L51 (-11.2419, -24.3967) -> (-32.734, 4.8)
  spline S139 degree 3 poles (-32.734, 4.8) (-32.9335, 5.0712) (-33.0179, 5.4104) (-32.9681, 5.7435) knots 0 0 0 0 1 1 1 1
  spline S140 degree 3 poles (-32.9681, 5.7435) (-32.9186, 6.0766) (-32.7393, 6.3767) (-32.4694, 6.578) knots 0 0 0 0 1 1 1 1
  spline S141 degree 3 poles (-32.4694, 6.578) (-32.2535, 6.7399) (-31.9905, 6.8273) (-31.7206, 6.8267) knots 0 0 0 0 1 1 1 1
  spline S142 degree 3 poles (-2.3571, 2.7813) (-2.3032, 2.7233) (-2.2381, 2.6767) (-2.1659, 2.6439) knots 0 0 0 0 1 1 1 1
  spline S143 degree 3 poles (-2.1659, 2.6439) (-2.0939, 2.6111) (-2.0158, 2.5931) (-1.9367, 2.5907) knots 0 0 0 0 1 1 1 1
  spline S144 degree 3 poles (-1.9367, 2.5907) (-1.8573, 2.5881) (-1.7785, 2.6016) (-1.7044, 2.6296) knots 0 0 0 0 1 1 1 1
  spline S145 degree 3 poles (-1.7044, 2.6296) (-1.6303, 2.6577) (-1.5626, 2.7003) (-1.5052, 2.7548) knots 0 0 0 0 1 1 1 1
  line L52 (-1.5052, 2.7548) -> (-1.4787, 2.7813)
  line L53 (-1.4787, 2.7813) -> (1.4793, 5.7155)
  spline S146 degree 3 poles (1.4793, 5.7155) (1.5952, 5.8229) (1.6643, 5.9716) (1.6717, 6.1293) knots 0 0 0 0 1 1 1 1
  spline S147 degree 3 poles (1.6717, 6.1293) (1.6791, 6.2872) (1.6243, 6.4418) (1.519, 6.5595) knots 0 0 0 0 1 1 1 1
  line L54 (1.519, 6.5595) -> (1.4793, 6.5992)
  spline S148 degree 3 poles (1.4793, 6.5992) (1.4285, 6.6577) (1.3663, 6.7053) (1.2968, 6.7394) knots 0 0 0 0 1 1 1 1
  spline S149 degree 3 poles (1.2968, 6.7394) (1.2272, 6.7735) (1.1512, 6.7934) (1.074, 6.7976) knots 0 0 0 0 1 1 1 1
  spline S150 degree 3 poles (1.074, 6.7976) (0.9964, 6.8021) (0.9192, 6.791) (0.8459, 6.7651) knots 0 0 0 0 1 1 1 1
  spline S151 degree 3 poles (0.8459, 6.7651) (0.7729, 6.7392) (0.7059, 6.6989) (0.6485, 6.6468) knots 0 0 0 0 1 1 1 1
  spline S152 degree 3 poles (0.6485, 6.6468) (0.6303, 6.6336) (0.6141, 6.6177) (0.6009, 6.5992) knots 0 0 0 0 1 1 1 1
  line L55 (0.6009, 6.5992) -> (-1.9179, 4.0909)
  line L56 (-1.9179, 4.0909) -> (-4.4341, 6.5992)
  spline S153 degree 3 poles (-4.4341, 6.5992) (-4.4913, 6.6579) (-4.5601, 6.704) (-4.6363, 6.7347) knots 0 0 0 0 1 1 1 1
  spline S154 degree 3 poles (-4.6363, 6.7347) (-4.7125, 6.7651) (-4.794, 6.7794) (-4.876, 6.7765) knots 0 0 0 0 1 1 1 1
  spline S155 degree 3 poles (-4.876, 6.7765) (-5.0398, 6.7759) (-5.1969, 6.7124) (-5.3152, 6.5992) knots 0 0 0 0 1 1 1 1
  spline S156 degree 3 poles (-5.3152, 6.5992) (-5.4311, 6.4918) (-5.5001, 6.3431) (-5.5075, 6.1854) knots 0 0 0 0 1 1 1 1
  spline S157 degree 3 poles (-5.5075, 6.1854) (-5.5149, 6.0274) (-5.4602, 5.8729) (-5.3549, 5.7552) knots 0 0 0 0 1 1 1 1
  line L57 (-5.3549, 5.7552) -> (-5.3152, 5.7155)
  line L58 (-5.3152, 5.7155) -> (-2.3571, 2.7813)
  spline S158 degree 3 poles (-2.3571, -0.4811) (-2.3032, -0.539) (-2.2381, -0.5857) (-2.1659, -0.6184) knots 0 0 0 0 1 1 1 1
  spline S159 degree 3 poles (-2.1659, -0.6184) (-2.0939, -0.6511) (-2.0158, -0.6692) (-1.9367, -0.6716) knots 0 0 0 0 1 1 1 1
  spline S160 degree 3 poles (-1.9367, -0.6716) (-1.8573, -0.6741) (-1.7785, -0.6608) (-1.7044, -0.6327) knots 0 0 0 0 1 1 1 1
  spline S161 degree 3 poles (-1.7044, -0.6327) (-1.6303, -0.6045) (-1.5626, -0.562) (-1.5052, -0.5075) knots 0 0 0 0 1 1 1 1
  line L59 (-1.5052, -0.5075) -> (-1.4787, -0.4811)
  line L60 (-1.4787, -0.4811) -> (1.4793, 2.4743)
  spline S162 degree 3 poles (1.4793, 2.4743) (1.5952, 2.5818) (1.6643, 2.7304) (1.6717, 2.8881) knots 0 0 0 0 1 1 1 1
  spline S163 degree 3 poles (1.6717, 2.8881) (1.6791, 3.0461) (1.6243, 3.2006) (1.519, 3.3184) knots 0 0 0 0 1 1 1 1
  line L61 (1.519, 3.3184) -> (1.4793, 3.3607)
  spline S164 degree 3 poles (1.4793, 3.3607) (1.428, 3.4184) (1.3658, 3.4655) (1.2962, 3.4993) knots 0 0 0 0 1 1 1 1
  spline S165 degree 3 poles (1.2962, 3.4993) (1.2266, 3.5329) (1.151, 3.5525) (1.0737, 3.557) knots 0 0 0 0 1 1 1 1
  spline S166 degree 3 poles (1.0737, 3.557) (0.9967, 3.5615) (0.9195, 3.5507) (0.8464, 3.525) knots 0 0 0 0 1 1 1 1
  spline S167 degree 3 poles (0.8464, 3.525) (0.7734, 3.4996) (0.7062, 3.4599) (0.6485, 3.4083) knots 0 0 0 0 1 1 1 1
  spline S168 degree 3 poles (0.6485, 3.4083) (0.6313, 3.3938) (0.6154, 3.3779) (0.6009, 3.3607) knots 0 0 0 0 1 1 1 1
  line L62 (0.6009, 3.3607) -> (-1.9179, 0.8524)
  line L63 (-1.9179, 0.8524) -> (-4.4341, 3.3607)
  spline S169 degree 3 poles (-4.4341, 3.3607) (-4.4913, 3.4194) (-4.5601, 3.4655) (-4.6363, 3.4962) knots 0 0 0 0 1 1 1 1
  spline S170 degree 3 poles (-4.6363, 3.4962) (-4.7125, 3.5266) (-4.794, 3.5409) (-4.876, 3.538) knots 0 0 0 0 1 1 1 1
  spline S171 degree 3 poles (-4.876, 3.538) (-5.0398, 3.5374) (-5.1969, 3.4739) (-5.3152, 3.3607) knots 0 0 0 0 1 1 1 1
  spline S172 degree 3 poles (-5.3152, 3.3607) (-5.4311, 3.2533) (-5.5001, 3.1046) (-5.5075, 2.9469) knots 0 0 0 0 1 1 1 1
  spline S173 degree 3 poles (-5.5075, 2.9469) (-5.5149, 2.7889) (-5.4602, 2.6344) (-5.3549, 2.5167) knots 0 0 0 0 1 1 1 1
  line L64 (-5.3549, 2.5167) -> (-5.3152, 2.4743)
  line L65 (-5.3152, 2.4743) -> (-2.3571, -0.4811)
  spline S174 degree 3 poles (-2.3571, -3.4867) (-2.3034, -3.5451) (-2.2386, -3.5923) (-2.1666, -3.6255) knots 0 0 0 0 1 1 1 1
  spline S175 degree 3 poles (-2.1666, -3.6255) (-2.0944, -3.6586) (-2.0166, -3.677) (-1.9373, -3.6797) knots 0 0 0 0 1 1 1 1
  spline S176 degree 3 poles (-1.9373, -3.6797) (-1.8579, -3.6825) (-1.779, -3.6694) (-1.7047, -3.6412) knots 0 0 0 0 1 1 1 1
  spline S177 degree 3 poles (-1.7047, -3.6412) (-1.6306, -3.6131) (-1.5629, -3.5704) (-1.5052, -3.5158) knots 0 0 0 0 1 1 1 1
  line L66 (-1.5052, -3.5158) -> (-1.4787, -3.4867)
  line L67 (-1.4787, -3.4867) -> (1.4793, -0.5287)
  spline S178 degree 3 poles (1.4793, -0.5287) (1.5952, -0.4109) (1.6603, -0.2522) (1.6603, -0.0868) knots 0 0 0 0 1 1 1 1
  spline S179 degree 3 poles (1.6603, -0.0868) (1.6603, 0.0785) (1.5952, 0.2372) (1.4793, 0.355) knots 0 0 0 0 1 1 1 1
  spline S180 degree 3 poles (1.4793, 0.355) (1.4222, 0.4136) (1.3539, 0.4601) (1.2785, 0.4919) knots 0 0 0 0 1 1 1 1
  spline S181 degree 3 poles (1.2785, 0.4919) (1.2031, 0.5237) (1.1219, 0.54) (1.0401, 0.54) knots 0 0 0 0 1 1 1 1
  spline S182 degree 3 poles (1.0401, 0.54) (0.9583, 0.54) (0.8771, 0.5237) (0.8017, 0.4919) knots 0 0 0 0 1 1 1 1
  spline S183 degree 3 poles (0.8017, 0.4919) (0.7263, 0.4601) (0.658, 0.4136) (0.6009, 0.355) knots 0 0 0 0 1 1 1 1
  line L68 (0.6009, 0.355) -> (-1.9179, -2.1532)
  line L69 (-1.9179, -2.1532) -> (-4.4341, 0.355)
  spline S184 degree 3 poles (-4.4341, 0.355) (-4.4915, 0.4132) (-4.5606, 0.4587) (-4.6368, 0.4888) knots 0 0 0 0 1 1 1 1
  spline S185 degree 3 poles (-4.6368, 0.4888) (-4.7127, 0.5189) (-4.7942, 0.5328) (-4.876, 0.5296) knots 0 0 0 0 1 1 1 1
  spline S186 degree 3 poles (-4.876, 0.5296) (-5.0392, 0.5299) (-5.1967, 0.4673) (-5.3152, 0.355) knots 0 0 0 0 1 1 1 1
  spline S187 degree 3 poles (-5.3152, 0.355) (-5.4308, 0.248) (-5.4999, 0.0999) (-5.5073, -0.0575) knots 0 0 0 0 1 1 1 1
  spline S188 degree 3 poles (-5.5073, -0.0575) (-5.5147, -0.2149) (-5.4599, -0.3689) (-5.3549, -0.4864) knots 0 0 0 0 1 1 1 1
  line L70 (-5.3549, -0.4864) -> (-5.3152, -0.5287)
  line L71 (-5.3152, -0.5287) -> (-2.3571, -3.4867)
  spline S189 degree 3 poles (-10.6704, 2.7813) (-10.618, 2.7236) (-10.5547, 2.6765) (-10.4841, 2.6431) knots 0 0 0 0 1 1 1 1
  spline S190 degree 3 poles (-10.4841, 2.6431) (-10.4137, 2.6101) (-10.3372, 2.591) (-10.2592, 2.5873) knots 0 0 0 0 1 1 1 1
  spline S191 degree 3 poles (-10.2592, 2.5873) (-10.1814, 2.5836) (-10.1034, 2.5952) (-10.0301, 2.6217) knots 0 0 0 0 1 1 1 1
  spline S192 degree 3 poles (-10.0301, 2.6217) (-9.9568, 2.6482) (-9.8893, 2.6889) (-9.8316, 2.7416) knots 0 0 0 0 1 1 1 1
  line L72 (-9.8316, 2.7416) -> (-9.7919, 2.7813)
  line L73 (-9.7919, 2.7813) -> (-6.8524, 5.7155)
  spline S193 degree 3 poles (-6.8524, 5.7155) (-6.7357, 5.8221) (-6.6656, 5.9708) (-6.6577, 6.1288) knots 0 0 0 0 1 1 1 1
  spline S194 degree 3 poles (-6.6577, 6.1288) (-6.6497, 6.2867) (-6.7045, 6.4415) (-6.8101, 6.5595) knots 0 0 0 0 1 1 1 1
  line L74 (-6.8101, 6.5595) -> (-6.8524, 6.5992)
  spline S195 degree 3 poles (-6.8524, 6.5992) (-6.9101, 6.6566) (-6.9786, 6.7021) (-7.054, 6.7325) knots 0 0 0 0 1 1 1 1
  spline S196 degree 3 poles (-7.054, 6.7325) (-7.1294, 6.763) (-7.2104, 6.778) (-7.2916, 6.7765) knots 0 0 0 0 1 1 1 1
  spline S197 degree 3 poles (-7.2916, 6.7765) (-7.4554, 6.7762) (-7.6128, 6.7127) (-7.7308, 6.5992) knots 0 0 0 0 1 1 1 1
  line L75 (-7.7308, 6.5992) -> (-10.2444, 4.0909)
  line L76 (-10.2444, 4.0909) -> (-12.7606, 6.5992)
  spline S198 degree 3 poles (-12.7606, 6.5992) (-12.8177, 6.6577) (-12.886, 6.7042) (-12.9614, 6.736) knots 0 0 0 0 1 1 1 1
  spline S199 degree 3 poles (-12.9614, 6.736) (-13.0371, 6.7677) (-13.118, 6.7841) (-13.1998, 6.7841) knots 0 0 0 0 1 1 1 1
  spline S200 degree 3 poles (-13.1998, 6.7841) (-13.2815, 6.7841) (-13.3628, 6.7677) (-13.4382, 6.736) knots 0 0 0 0 1 1 1 1
  spline S201 degree 3 poles (-13.4382, 6.736) (-13.5136, 6.7042) (-13.5818, 6.6577) (-13.639, 6.5992) knots 0 0 0 0 1 1 1 1
  spline S202 degree 3 poles (-13.639, 6.5992) (-13.7557, 6.4817) (-13.821, 6.323) (-13.821, 6.1573) knots 0 0 0 0 1 1 1 1
  spline S203 degree 3 poles (-13.821, 6.1573) (-13.821, 5.9917) (-13.7557, 5.833) (-13.639, 5.7155) knots 0 0 0 0 1 1 1 1
  line L77 (-13.639, 5.7155) -> (-10.6704, 2.7813)
  spline S204 degree 3 poles (-10.6704, -0.4811) (-10.618, -0.5389) (-10.5547, -0.5858) (-10.4841, -0.619) knots 0 0 0 0 1 1 1 1
  spline S205 degree 3 poles (-10.4841, -0.619) (-10.4134, -0.6523) (-10.3372, -0.6714) (-10.2592, -0.6751) knots 0 0 0 0 1 1 1 1
  spline S206 degree 3 poles (-10.2592, -0.6751) (-10.1814, -0.6787) (-10.1034, -0.667) (-10.0301, -0.6405) knots 0 0 0 0 1 1 1 1
  spline S207 degree 3 poles (-10.0301, -0.6405) (-9.9565, -0.614) (-9.8893, -0.5733) (-9.8316, -0.5208) knots 0 0 0 0 1 1 1 1
  line L78 (-9.8316, -0.5208) -> (-9.7919, -0.4811)
  line L79 (-9.7919, -0.4811) -> (-6.8524, 2.4743)
  spline S208 degree 3 poles (-6.8524, 2.4743) (-6.7389, 2.5897) (-6.6751, 2.745) (-6.6751, 2.9069) knots 0 0 0 0 1 1 1 1
  spline S209 degree 3 poles (-6.6751, 2.9069) (-6.6751, 3.0689) (-6.7389, 3.2242) (-6.8524, 3.3395) knots 0 0 0 0 1 1 1 1
  spline S210 degree 3 poles (-6.8524, 3.3395) (-6.9104, 3.3983) (-6.9797, 3.4443) (-7.0561, 3.4753) knots 0 0 0 0 1 1 1 1
  spline S211 degree 3 poles (-7.0561, 3.4753) (-7.1326, 3.5062) (-7.2144, 3.5213) (-7.2969, 3.5194) knots 0 0 0 0 1 1 1 1
  spline S212 degree 3 poles (-7.2969, 3.5194) (-7.4607, 3.5192) (-7.6181, 3.4557) (-7.7361, 3.3422) knots 0 0 0 0 1 1 1 1
  line L80 (-7.7361, 3.3422) -> (-10.2497, 0.8339)
  line L81 (-10.2497, 0.8339) -> (-12.7659, 3.3422)
  spline S213 degree 3 poles (-12.7659, 3.3422) (-12.8717, 3.4586) (-13.0193, 3.5284) (-13.1765, 3.5364) knots 0 0 0 0 1 1 1 1
  spline S214 degree 3 poles (-13.1765, 3.5364) (-13.3337, 3.5443) (-13.4876, 3.4898) (-13.6046, 3.3845) knots 0 0 0 0 1 1 1 1
  line L82 (-13.6046, 3.3845) -> (-13.6443, 3.3422)
  spline S215 degree 3 poles (-13.6443, 3.3422) (-13.7022, 3.2845) (-13.7483, 3.2157) (-13.7797, 3.14) knots 0 0 0 0 1 1 1 1
  spline S216 degree 3 poles (-13.7797, 3.14) (-13.811, 3.0646) (-13.8271, 2.9834) (-13.8271, 2.9016) knots 0 0 0 0 1 1 1 1
  spline S217 degree 3 poles (-13.8271, 2.9016) (-13.8271, 2.8199) (-13.811, 2.7387) (-13.7797, 2.6632) knots 0 0 0 0 1 1 1 1
  spline S218 degree 3 poles (-13.7797, 2.6632) (-13.7483, 2.5876) (-13.7022, 2.5188) (-13.6443, 2.4611) knots 0 0 0 0 1 1 1 1
  line L83 (-13.6443, 2.4611) -> (-10.6704, -0.4811)
  spline S219 degree 3 poles (-10.6704, -3.4867) (-10.6185, -3.545) (-10.5553, -3.5924) (-10.4849, -3.6261) knots 0 0 0 0 1 1 1 1
  spline S220 degree 3 poles (-10.4849, -3.6261) (-10.4142, -3.6598) (-10.3378, -3.6792) (-10.26, -3.6832) knots 0 0 0 0 1 1 1 1
  spline S221 degree 3 poles (-10.26, -3.6832) (-10.1819, -3.6871) (-10.1039, -3.6755) (-10.0303, -3.6491) knots 0 0 0 0 1 1 1 1
  spline S222 degree 3 poles (-10.0303, -3.6491) (-9.9568, -3.6226) (-9.8893, -3.5818) (-9.8316, -3.5291) knots 0 0 0 0 1 1 1 1
  line L84 (-9.8316, -3.5291) -> (-9.7919, -3.4867)
  line L85 (-9.7919, -3.4867) -> (-6.8524, -0.5287)
  spline S223 degree 3 poles (-6.8524, -0.5287) (-6.7357, -0.422) (-6.6656, -0.2734) (-6.6577, -0.1154) knots 0 0 0 0 1 1 1 1
  spline S224 degree 3 poles (-6.6577, -0.1154) (-6.6497, 0.0427) (-6.7045, 0.1974) (-6.8101, 0.3153) knots 0 0 0 0 1 1 1 1
  spline S225 degree 3 poles (-6.8101, 0.3153) (-6.823, 0.3299) (-6.8371, 0.3432) (-6.8524, 0.355) knots 0 0 0 0 1 1 1 1
  spline S226 degree 3 poles (-6.8524, 0.355) (-6.9101, 0.4121) (-6.9789, 0.4569) (-7.0543, 0.4869) knots 0 0 0 0 1 1 1 1
  spline S227 degree 3 poles (-7.0543, 0.4869) (-7.1297, 0.5169) (-7.2104, 0.5314) (-7.2916, 0.5296) knots 0 0 0 0 1 1 1 1
  spline S228 degree 3 poles (-7.2916, 0.5296) (-7.4551, 0.5299) (-7.6123, 0.4673) (-7.7308, 0.355) knots 0 0 0 0 1 1 1 1
  line L86 (-7.7308, 0.355) -> (-10.1968, -2.1532)
  line L87 (-10.1968, -2.1532) -> (-12.7129, 0.355)
  spline S229 degree 3 poles (-12.7129, 0.355) (-12.7701, 0.4136) (-12.8383, 0.4601) (-12.9138, 0.4919) knots 0 0 0 0 1 1 1 1
  spline S230 degree 3 poles (-12.9138, 0.4919) (-12.9894, 0.5237) (-13.0704, 0.54) (-13.1521, 0.54) knots 0 0 0 0 1 1 1 1
  spline S231 degree 3 poles (-13.1521, 0.54) (-13.2339, 0.54) (-13.3151, 0.5237) (-13.3905, 0.4919) knots 0 0 0 0 1 1 1 1
  spline S232 degree 3 poles (-13.3905, 0.4919) (-13.4659, 0.4601) (-13.5342, 0.4136) (-13.5914, 0.355) knots 0 0 0 0 1 1 1 1
  spline S233 degree 3 poles (-13.5914, 0.355) (-13.708, 0.2375) (-13.7734, 0.0787) (-13.7734, -0.0868) knots 0 0 0 0 1 1 1 1
  spline S234 degree 3 poles (-13.7734, -0.0868) (-13.7734, -0.2524) (-13.708, -0.4112) (-13.5914, -0.5287) knots 0 0 0 0 1 1 1 1
  line L88 (-13.5914, -0.5287) -> (-10.6704, -3.4867)
  spline S235 degree 3 poles (-18.9783, 2.7813) (-18.9259, 2.7236) (-18.8626, 2.6765) (-18.792, 2.6431) knots 0 0 0 0 1 1 1 1
  spline S236 degree 3 poles (-18.792, 2.6431) (-18.7216, 2.6101) (-18.6452, 2.591) (-18.5671, 2.5873) knots 0 0 0 0 1 1 1 1
  spline S237 degree 3 poles (-18.5671, 2.5873) (-18.4893, 2.5836) (-18.4113, 2.5952) (-18.338, 2.6217) knots 0 0 0 0 1 1 1 1
  spline S238 degree 3 poles (-18.338, 2.6217) (-18.2647, 2.6482) (-18.1972, 2.6889) (-18.1395, 2.7416) knots 0 0 0 0 1 1 1 1
  line L89 (-18.1395, 2.7416) -> (-18.0999, 2.7812)
  line L90 (-18.0999, 2.7812) -> (-15.1656, 5.7049)
  spline S239 degree 3 poles (-15.1656, 5.7049) (-15.0489, 5.8115) (-14.9788, 5.9602) (-14.9709, 6.1182) knots 0 0 0 0 1 1 1 1
  spline S240 degree 3 poles (-14.9709, 6.1182) (-14.963, 6.2761) (-15.0177, 6.4309) (-15.1233, 6.5489) knots 0 0 0 0 1 1 1 1
  line L91 (-15.1233, 6.5489) -> (-15.1656, 6.5886)
  spline S241 degree 3 poles (-15.1656, 6.5886) (-15.2167, 6.6471) (-15.2786, 6.6947) (-15.3482, 6.7288) knots 0 0 0 0 1 1 1 1
  spline S242 degree 3 poles (-15.3482, 6.7288) (-15.418, 6.763) (-15.4937, 6.7828) (-15.571, 6.787) knots 0 0 0 0 1 1 1 1
  spline S243 degree 3 poles (-15.571, 6.787) (-15.6485, 6.7915) (-15.726, 6.7804) (-15.799, 6.7545) knots 0 0 0 0 1 1 1 1
  spline S244 degree 3 poles (-15.799, 6.7545) (-15.8721, 6.7286) (-15.9393, 6.6884) (-15.9964, 6.6362) knots 0 0 0 0 1 1 1 1
  spline S245 degree 3 poles (-15.9964, 6.6362) (-16.0136, 6.6217) (-16.0295, 6.6058) (-16.044, 6.5886) knots 0 0 0 0 1 1 1 1
  line L92 (-16.044, 6.5886) -> (-18.5602, 4.0804)
  line L93 (-18.5602, 4.0804) -> (-21.0526, 6.6151)
  spline S246 degree 3 poles (-21.0526, 6.6151) (-21.1098, 6.6727) (-21.1783, 6.718) (-21.254, 6.7476) knots 0 0 0 0 1 1 1 1
  spline S247 degree 3 poles (-21.254, 6.7476) (-21.3296, 6.7773) (-21.4106, 6.7905) (-21.4918, 6.787) knots 0 0 0 0 1 1 1 1
  spline S248 degree 3 poles (-21.4918, 6.787) (-21.6553, 6.7902) (-21.8133, 6.7283) (-21.931, 6.6151) knots 0 0 0 0 1 1 1 1
  spline S249 degree 3 poles (-21.931, 6.6151) (-21.9892, 6.5616) (-22.0361, 6.4971) (-22.0691, 6.4256) knots 0 0 0 0 1 1 1 1
  spline S250 degree 3 poles (-22.0691, 6.4256) (-22.1025, 6.3539) (-22.121, 6.2764) (-22.1244, 6.1976) knots 0 0 0 0 1 1 1 1
  spline S251 degree 3 poles (-22.1244, 6.1976) (-22.1276, 6.1187) (-22.1152, 6.0399) (-22.0879, 5.9658) knots 0 0 0 0 1 1 1 1
  spline S252 degree 3 poles (-22.0879, 5.9658) (-22.0607, 5.8917) (-22.0189, 5.8237) (-21.9654, 5.7657) knots 0 0 0 0 1 1 1 1
  spline S253 degree 3 poles (-21.9654, 5.7657) (-21.9554, 5.7531) (-21.9437, 5.7414) (-21.931, 5.7314) knots 0 0 0 0 1 1 1 1
  line L94 (-21.931, 5.7314) -> (-18.9783, 2.7813)
  spline S254 degree 3 poles (-18.9783, -0.4811) (-18.9259, -0.5389) (-18.8626, -0.5858) (-18.792, -0.619) knots 0 0 0 0 1 1 1 1
  spline S255 degree 3 poles (-18.792, -0.619) (-18.7216, -0.6523) (-18.6452, -0.6714) (-18.5671, -0.6751) knots 0 0 0 0 1 1 1 1
  spline S256 degree 3 poles (-18.5671, -0.6751) (-18.4893, -0.6787) (-18.4113, -0.667) (-18.338, -0.6405) knots 0 0 0 0 1 1 1 1
  spline S257 degree 3 poles (-18.338, -0.6405) (-18.2647, -0.614) (-18.1972, -0.5733) (-18.1395, -0.5208) knots 0 0 0 0 1 1 1 1
  line L95 (-18.1395, -0.5208) -> (-18.0999, -0.4811)
  line L96 (-18.0999, -0.4811) -> (-15.1656, 2.4743)
  spline S258 degree 3 poles (-15.1656, 2.4743) (-15.0489, 2.581) (-14.9788, 2.7297) (-14.9709, 2.8876) knots 0 0 0 0 1 1 1 1
  spline S259 degree 3 poles (-14.9709, 2.8876) (-14.963, 3.0456) (-15.0177, 3.2003) (-15.1233, 3.3184) knots 0 0 0 0 1 1 1 1
  spline S260 degree 3 poles (-15.1233, 3.3184) (-15.136, 3.3337) (-15.1503, 3.348) (-15.1656, 3.3607) knots 0 0 0 0 1 1 1 1
  spline S261 degree 3 poles (-15.1656, 3.3607) (-15.222, 3.4178) (-15.2892, 3.4631) (-15.3633, 3.494) knots 0 0 0 0 1 1 1 1
  spline S262 degree 3 poles (-15.3633, 3.494) (-15.4371, 3.525) (-15.5167, 3.5411) (-15.5969, 3.5411) knots 0 0 0 0 1 1 1 1
  spline S263 degree 3 poles (-15.5969, 3.5411) (-15.6771, 3.5411) (-15.7567, 3.525) (-15.8305, 3.494) knots 0 0 0 0 1 1 1 1
  spline S264 degree 3 poles (-15.8305, 3.494) (-15.9046, 3.4631) (-15.9718, 3.4178) (-16.0282, 3.3607) knots 0 0 0 0 1 1 1 1
  line L97 (-16.0282, 3.3607) -> (-16.044, 3.3607)
  line L98 (-16.044, 3.3607) -> (-18.5602, 0.8524)
  line L99 (-18.5602, 0.8524) -> (-21.0526, 3.3607)
  spline S265 degree 3 poles (-21.0526, 3.3607) (-21.1092, 3.4194) (-21.1778, 3.4655) (-21.2534, 3.4959) knots 0 0 0 0 1 1 1 1
  spline S266 degree 3 poles (-21.2534, 3.4959) (-21.3291, 3.5266) (-21.4103, 3.5409) (-21.4918, 3.538) knots 0 0 0 0 1 1 1 1
  spline S267 degree 3 poles (-21.4918, 3.538) (-21.6556, 3.5382) (-21.8133, 3.4747) (-21.931, 3.3607) knots 0 0 0 0 1 1 1 1
  spline S268 degree 3 poles (-21.931, 3.3607) (-22.048, 3.2541) (-22.1178, 3.1054) (-22.1258, 2.9474) knots 0 0 0 0 1 1 1 1
  spline S269 degree 3 poles (-22.1258, 2.9474) (-22.1337, 2.7895) (-22.0789, 2.6347) (-21.9734, 2.5167) knots 0 0 0 0 1 1 1 1
  spline S270 degree 3 poles (-21.9734, 2.5167) (-21.9734, 2.5008) (-21.9442, 2.4876) (-21.931, 2.4743) knots 0 0 0 0 1 1 1 1
  line L100 (-21.931, 2.4743) -> (-18.9783, -0.4811)
  spline S271 degree 3 poles (-18.9783, -3.4867) (-18.9264, -3.545) (-18.8632, -3.5924) (-18.7928, -3.6261) knots 0 0 0 0 1 1 1 1
  spline S272 degree 3 poles (-18.7928, -3.6261) (-18.7222, -3.6598) (-18.6457, -3.6792) (-18.5679, -3.6832) knots 0 0 0 0 1 1 1 1
  spline S273 degree 3 poles (-18.5679, -3.6832) (-18.4898, -3.6871) (-18.4118, -3.6755) (-18.3382, -3.6491) knots 0 0 0 0 1 1 1 1
  spline S274 degree 3 poles (-18.3382, -3.6491) (-18.2647, -3.6226) (-18.1972, -3.5818) (-18.1395, -3.5291) knots 0 0 0 0 1 1 1 1
  line L101 (-18.1395, -3.5291) -> (-18.0999, -3.4867)
  line L102 (-18.0999, -3.4867) -> (-15.1656, -0.5287)
  spline S275 degree 3 poles (-15.1656, -0.5287) (-15.0489, -0.4112) (-14.9836, -0.2524) (-14.9836, -0.0868) knots 0 0 0 0 1 1 1 1